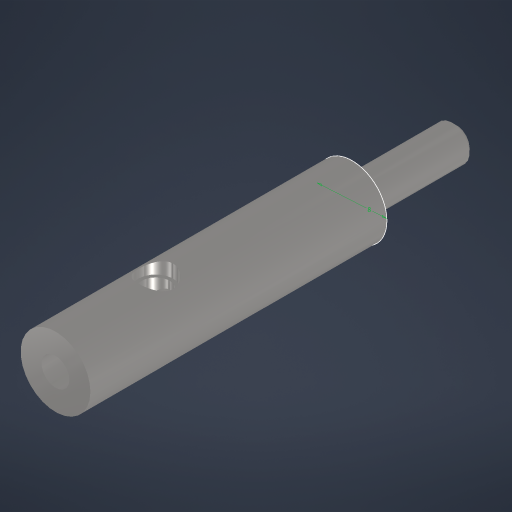
# Autodesk Inventor part: KURBELWELLE PART 7
Saved by Autodesk Inventor 2023 (Build 270158000, 158)
## iProperties
Created: 2020-07-02
Part Number: KURBELWELLE PART 7
Material: Stainless Steel
Document SubType Name: Modeling
Designer: Smit Ambardekar
Density: 8 g/cm^3
Appearance: Semi-Polished
Author: Smit Ambardekar
Autodesk Inventor part; units mm, degrees
sketch "Sketch1" plane through (0, 0, 0) normal (0, 0, 1) x (1, 0, 0)
  circle A0 centre (0, 0) radius 4
  dimension "d0" = 8
  constraints: 1 centre point, 1 coincident
  measures "d0" diameter of A0
extrude "Extrusion1" add sketch "Sketch1" along normal blind 34
sketch "Sketch2" plane through (0, 0, 0) normal (0, 0, -1) x (-1, 0, 0)
  circle A0 centre (0, 0) radius 2
  dimension "d3" = 4
  constraints: 1 centre point, 1 coincident
  measures "d3" diameter of A0
extrude "Extrusion2" add sketch "Sketch2" along normal blind 12
chamfer "Chamfer1" distance 0.5 angle 45 1 edges at (2, 0, -12)
sketch "Sketch3" plane through (0, 0, 34) normal (0, 0, 1) x (1, 0, 0)
  line L0 (0, 0) -> (0, 4)
  circle A0 centre (0, 0) radius 4 projected
  constraints: 2 end point, 1 vertical, 1 vertical alignment, 1 other
hole "Hole1" at (0, 0, 34) direction (0, 0, -1) diameter 3.2 depth 14 tip angle 118
ref_plane "Work Plane1" through (0, 4, 34) normal (0, 1, 0) x (-1, 0, 0)
ref_plane "Work Plane2" through (0, 0, 0) normal (1, 0, 0) x (0, 1, 0)
sketch "Sketch5" plane through (0, 0, 0) normal (1, 0, 0) x (0, 1, 0)
  line L0 (-4, 0) -> (-4, 34) projected
  line L1 (-4, 24.5) -> (-2.5, 24.5)
  line L2 (-2.5, 24.5) -> (-2.5, 12.5)
  line L3 (-2.5, 12.5) -> (-4, 12.5)
  line L4 (-4, 12.5) -> (-4, 24.5)
  line L5 (4, 34) -> (-4, 34) projected
  point P0 (0, 0)
  dimension "d19" = 12
  dimension "d20" = 9.5
  dimension "d21" = 1.5
  constraints: 8 end point, 2 parallel, 1 horizontal, 1 perpendicular, 1 point on line
  measures "d19" distance of L1.end L2.end
  measures "d20" distance between parallel lines of L5 L1
  measures "d21" distance of L2.end L3.end
extrude "Extrusion3" cut sketch "Sketch5" along normal mid plane 100
ref_plane "Work Plane3" through (0, 4, 0) normal (0, 1, 0) x (-1, 0, 0)
sketch "Sketch6" plane through (0, 4, 0) normal (0, 1, 0) x (-1, 0, 0)
  line L0 (4, 34) -> (-4, 34) projected
  line L1 (0, 34) -> (0, 22.5)
  point P0 (0, 0)
  dimension "d25" = 11.5
  constraints: 2 end point, 1 midpoint, 1 vertical
  measures "d25" distance of L1.start L1.end
hole "Hole2" at (0, 4, 22.5) direction (0, -1, 0) diameter 4 depth 1.5
hole "Hole3" at (0, 4, 22.5) direction (0, -1, 0) diameter 3.2 depth 4 tip angle 118
body "Solid1"
